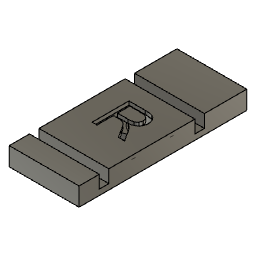
LEDHoldingMechanismBinderR (Autodesk Fusion 360 design; units mm, degrees)
Autodesk Fusion 360 part; units mm, degrees
sketch "Skizze1" plane through (0, 0, 0) normal (0, 0, 1) x (1, 0, 0)
  line L0 (9.75, 22.8) -> (-9.75, 22.8)
  line L1 (-9.75, 22.8) -> (-9.75, -22.8)
  line L2 (-9.75, -22.8) -> (9.75, -22.8)
  line L3 (9.75, -22.8) -> (9.75, 22.8)
  line L4 (9.75, 22.8) -> (-9.75, -22.8) construction
  line L5 (-9.75, 22.8) -> (9.75, -22.8) construction
  dimension "d1" = 19.5
  dimension "d2" = 45.6
  constraint horizontal L0
  constraint perpendicular L0 L1
  constraint parallel L0 L2
  constraint parallel L1 L3
  constraint coincident L4 origin
  constraint coincident L5 origin
  measures "d1" distance of L1.end L2.end
  measures "d2" distance of L0.end L1.end
extrude "Extrusion1" add sketch "Skizze1" along normal blind 5
sketch "Skizze2" plane through (0, 0, 5) normal (0, 0, 1) x (-1, 0, 0)
  line L0 (-9.75, 22.8) -> (-9.75, -22.8)
  line L1 (-9.75, -22.8) -> (9.75, -22.8)
  line L2 (9.75, -22.8) -> (9.75, 22.8)
  line L3 (9.75, 22.8) -> (-9.75, 22.8)
  line L4 (9.75, 22.8) -> (-9.75, 22.8)
  line L5 (-9.75, 22.8) -> (-9.75, 17.05)
  line L6 (-9.75, 17.05) -> (9.75, 17.05)
  line L7 (9.75, 17.05) -> (9.75, 22.8)
  line L8 (-9.75, -22.8) -> (9.75, -22.8)
  line L9 (9.75, -22.8) -> (9.75, -11.05)
  line L10 (9.75, -11.05) -> (-9.75, -11.05)
  line L11 (-9.75, -11.05) -> (-9.75, -22.8)
  dimension "d5" = 5.75
  dimension "d6" = 11.75
  constraint horizontal L4
  constraint vertical L5
  constraint horizontal L6
  constraint vertical L7
  constraint coincident L2.end L3.start
  constraint horizontal L8
  constraint vertical L9
  constraint horizontal L10
  constraint vertical L11
  constraint coincident L0.end L1.start
  measures "d5" distance of L2.end L6.end
  measures "d6" distance of L0.end L10.end
extrude "Extrusion2" cut sketch "Skizze2" against normal blind 3.5 contours L0 L2 L6 L10
sketch "Skizze4" plane through (0, 0, 1.5) normal (0, 0, 1) x (-1, 0, 0)
  line L0 (-9.75, 17.05) -> (-9.75, -11.05)
  line L1 (-9.75, -11.05) -> (9.75, -11.05)
  line L2 (9.75, -11.05) -> (9.75, 17.05)
  line L3 (9.75, 17.05) -> (-9.75, 17.05)
  line L4 (9.75, 14.7) -> (-9.75, 14.7)
  line L5 (-9.75, 14.7) -> (-9.75, -8.7)
  line L6 (-9.75, -8.7) -> (9.75, -8.7)
  line L7 (9.75, -8.7) -> (9.75, 14.7)
  line L8 (9.75, 14.7) -> (-9.75, -8.7) construction
  line L9 (-9.75, 14.7) -> (9.75, -8.7) construction
  point P0 (0, 3)
  dimension "d11" = 19.5
  dimension "d12" = 23.4
  constraint horizontal L4
  constraint perpendicular L4 L5
  constraint parallel L4 L6
  constraint parallel L5 L7
  constraint coincident L8 P0
  constraint coincident L9 P0
  measures "d11" distance of L5.end L6.end
  measures "d12" distance of L4.end L5.end
extrude "Extrusion3" add sketch "Skizze4" along normal blind 3.5 contours L0 L2 L4 L5 L6 L7
sketch "Skizze5" plane through (0, 0, 0) normal (0, 0, -1) x (1, 0, 0)
  line L0 (9.75, -22.8) -> (9.75, 22.8)
  line L1 (9.75, 22.8) -> (-9.75, 22.8)
  line L2 (-9.75, 22.8) -> (-9.75, -22.8)
  line L3 (-9.75, -22.8) -> (9.75, -22.8)
  circle A0 centre (4, -2.5) radius 5.125
  circle A1 centre (4, 8) radius 5.125
  dimension "d15" = 10.25
  dimension "d16" = 10.25
  measures "d15" diameter of A0
  measures "d16" diameter of A1
extrude "Extrusion4" cut sketch "Skizze5" against normal up to surface (4 mm away) contours A0 | A1
move_face "Flächen versetzen1" offset -0.25 2 faces at (-3.25, 11.05, 3.8333) (3.25, -17.05, 3.8333)
sketch "Skizze7" plane through (0, 0, 5) normal (0, 0, 1) x (-1, 0, 0)
  line L0 (9.75, -8.7) -> (9.75, 14.7)
  line L1 (-9.75, 14.7) -> (-9.75, -8.7)
  line L2 (4, 10) -> (-5, 10) construction
  line L3 (-5, 10) -> (-5, -4) construction
  line L4 (-5, -4) -> (4, -4) construction
  line L5 (4, -4) -> (4, 10) construction
  line L6 (9.75, 14.7) -> (-9.75, 14.7)
  line L7 (-9.75, -8.7) -> (9.75, -8.7)
  dimension "d23" = 10
  text T0 "R" font "Arial" height 10 align left top in box 9 x 14 at (4, 10) x (-1, 0) y (0, -1) spacing 1
extrude "Extrusion6" cut sketch "Skizze7" against normal blind 1 text T0
move_face "Flächen versetzen2" offset -0.5 1 faces at (9.75, 18.9667, 2.1667)
